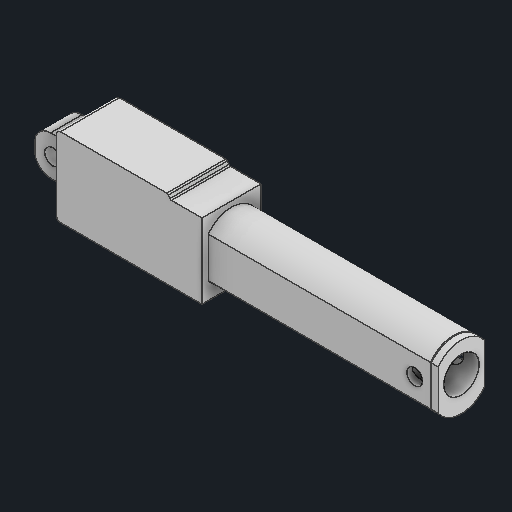
# Autodesk Inventor part: LA-T8-1215-50 105-64 Body
Saved by Autodesk Inventor 2025.2 (Build 292293000, 293)
## iProperties
Created: 2025-08-13
Part Number: LA-T8-1215-50 105-64 Body
Material: Generic
Document SubType Name: Modeling
Designer: valer
Density: 1 g/cm^3
Appearance: Default
Author: valer
Autodesk Inventor part; units mm, degrees
ref_plane "YZ Plane" through (0, 0, 0) normal (1, 0, 0) x (0, 1, 0)
ref_plane "XZ Plane" through (0, 0, 0) normal (0, 1, 0) x (-1, 0, 0)
ref_plane "XY Plane" through (0, 0, 0) normal (0, 0, 1) x (1, 0, 0)
sketch "Base" plane through (0, 0, 0) normal (0, 0, 1) x (1, 0, 0)
  circle A0 centre (0, 0) radius 2
  line L0 (-4.5, 5) -> (4.5, 5)
  line L1 (4.5, 5) -> (4.5, -5)
  line L2 (4.5, -5) -> (-4.5, -5)
  line L3 (-4.5, -5) -> (-4.5, 5)
  line L4 (4.5, 0) -> (-4.5, 0) construction
  line L5 (4.5, 10) -> (41.5, 10)
  line L6 (41.5, 10) -> (41.5, -10)
  line L7 (41.5, -10) -> (4.5, -10)
  line L8 (4.5, -10) -> (4.5, 10)
  dimension "d0" = 4
  dimension "d1" = 10
  dimension "d2" = 9
  dimension "d3" = 20
  dimension "d4" = 37
  constraints: 18 end point, 4 midpoint, 4 parallel, 2 coincident, 2 horizontal, 2 perpendicular, 1 centre point
  measures "d0" diameter of A0
  measures "d1" distance of L2.end L0.start
  measures "d2" distance of L0.start L0.end
  measures "d3" distance of L7.end L5.start
  measures "d4" distance of L5.start L5.end
extrude "Extrusion1" add sketch "Base" along normal mid plane 8 contours L0 L1 L2 L3
extrude "Extrusion2" add sketch "Base" along normal mid plane 15 contours L8 L5 L6 L7 L1
fillet "Fillet1" radius 4 2 edges at (-4.5, -5, 0) (-4.5, 5, 0)
fillet "Fillet2" radius 1 2 edges at (4.5, 10, 0) (4.5, -10, 0)
sketch "Sketch2" plane through (0, 0, 7.5) normal (0, 0, 1) x (1, 0, 0)
  arc A0 (4.5, -9) -> (5.5, -10) centre (5.5, -9) ccw projected
  line L0 (5.5, -10) -> (41.5, -10) projected
  line L1 (41.5, -10) -> (41.5, 10) projected
  line L2 (41.5, 10) -> (5.5, 10) projected
  arc A1 (5.5, 10) -> (4.5, 9) centre (5.5, 9) ccw projected
  line L3 (4.5, 9) -> (4.5, -9) projected
  line L4 (32.7998, 10) -> (33.5, 9)
  line L5 (33.5, 9) -> (41.5, 9)
  line L6 (41.5, -10) -> (41.5, 10) projected
  line L7 (41.5, 10) -> (5.5, 10) projected
  point P0 (0, 0)
  dimension "d11" = 1
  dimension "d12" = 8
  dimension "d13" = 125
  constraints: 4 end point, 2 point on line, 1 parallel, 1 perpendicular
  measures "d11" distance between parallel lines of L2 L5
  measures "d12" distance of L5.end L4.end
  measures "d13" angle of L5 L4
extrude "Extrusion3" cut sketch "Sketch2" against normal up to surface (15 mm away) contours L5 L4 L2 L1
fillet "Fillet3" radius 0.5 2 edges at (32.7998, 10, 0) (33.5, 9, 0)
sketch "Sketch3" plane through (41.5, -10, 7.5) normal (1, 0, 0) x (0, 0, -1)
  line L0 (15, 19) -> (0, 19) construction
  line L1 (7.5, 19) -> (7.5, 0) construction
  line L2 (0, 0) -> (15, 0) construction
  line L3 (1.625, 14.625) -> (13.375, 14.625) construction
  line L4 (13.375, 14.625) -> (13.375, 4.375)
  line L5 (13.375, 4.375) -> (1.625, 4.375) construction
  line L6 (1.625, 4.375) -> (1.625, 14.625)
  line L7 (0, 0) -> (0, 19) construction
  line L8 (0, 9.5) -> (15, 9.5) construction
  line L9 (15, 19) -> (15, 0) construction
  arc A0 (13.375, 14.625) -> (1.625, 14.625) centre (7.5, 10.3724) ccw
  arc A1 (1.625, 4.375) -> (13.375, 4.375) centre (7.5, 8.6276) ccw
  point P0 (7.5, 10)
  point P1 (7.5, 14.625)
  point P2 (1.625, 9.5)
  point P3 (7.5, 17.625)
  point P4 (7.5, 1.375)
  dimension "d17" = 11.75
  dimension "d18" = 3
  dimension "d21" = 16.25
  constraints: 12 end point, 6 midpoint, 6 point on circle, 2 centre point, 2 parallel, 2 point on line, 1 horizontal, 1 perpendicular, 1 symmetric about line, 1 other
  measures "d17" distance of L3.start L3.end
  measures "d18" distance of point (7.5, 14.625) point (7.5, 17.625)
  measures "d21" distance of point (7.5, 1.375) point (7.5, 17.625)
extrude "Extrusion4" add sketch "Sketch3" along normal blind 56.5
sketch "Sketch4" plane through (98, -10, 7.5) normal (1, 0, 0) x (0, 0, -1)
  line L0 (13.375, 4.375) -> (13.375, 14.625) projected
  arc A0 (13.375, 14.625) -> (1.625, 14.625) centre (7.5, 10.3724) ccw projected
  line L1 (1.625, 14.625) -> (1.625, 4.375) projected
  arc A1 (1.625, 4.375) -> (13.375, 4.375) centre (7.5, 8.6276) ccw projected
  arc A2 (12.875, 14.4598) -> (2.125, 14.4598) centre (7.5, 10.3724) ccw
  line L2 (12.875, 14.4598) -> (12.875, 4.5402)
  arc A3 (2.125, 4.5402) -> (12.875, 4.5402) centre (7.5, 8.6276) ccw
  line L3 (2.125, 4.5402) -> (2.125, 14.4598)
  point P0 (7.5, 10)
  dimension "d22" = 0.5
  constraints: 4 end point, 4 point on circle, 2 centre point, 3 other
  measures "d22" radial gap between concentric circles of A0 A2
extrude "Extrusion5" add sketch "Sketch4" along normal blind 0.25 contours L2 A3 L3 A2
sketch "Sketch5" plane through (98.25, -10, 7.5) normal (1, 0, 0) x (0, 0, -1)
  arc A0 (13.375, 14.625) -> (1.625, 14.625) centre (7.5, 10.3724) ccw projected
  line L0 (1.625, 14.625) -> (1.625, 4.375) projected
  arc A1 (1.625, 4.375) -> (13.375, 4.375) centre (7.5, 8.6276) ccw projected
  line L1 (13.375, 4.375) -> (13.375, 14.625) projected
  point P0 (7.5, 10)
extrude "Extrusion6" add sketch "Sketch5" along normal blind 1.75
sketch "Sketch6" plane through (100, -10, 7.5) normal (1, 0, 0) x (0, 0, -1)
  circle A0 centre (7.5, 10) radius 4.5
  dimension "d27" = 9
  constraints: 1 centre point, 1 coincident
  measures "d27" diameter of A0
extrude "Extrusion7" cut sketch "Sketch6" against normal blind 50
sketch "Sketch7" plane through (41.5, -5.625, 5.875) normal (0, 0, 1) x (1, 0, 0)
  line L0 (58.5, 0) -> (58.5, 10.25) projected
  line L1 (58.5, 5.125) -> (54.5, 5.125) construction
  circle A0 centre (52.5, 5.125) radius 2
  line L2 (52.5, 5.125) -> (54.5, 5.125) construction
  point P0 (-41.5, 5.625)
  dimension "d31" = 4
  dimension "d30" = 4
  constraints: 4 end point, 1 collinear, 1 horizontal, 1 horizontal alignment, 1 midpoint, 2 other
  measures "d30" distance of L1.start L1.end
extrude "Extrusion8" cut sketch "Sketch7" against normal through all
body "Solid1"
